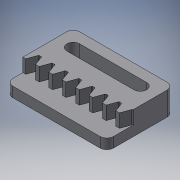
# Autodesk Inventor part: RackTest
Saved by Autodesk Inventor 2019 (Build 230136000, 136)
## iProperties
Created: 2019-07-15
Part Number: RackTest
Material: Generic
Document SubType Name: Modeling
Designer: aorfi
Density: 1 g/cm^3
Appearance: Default
Author: aorfi
Autodesk Inventor part; units mm, degrees
ref_plane "YZ Plane" through (0, 0, 0) normal (1, 0, 0) x (0, 1, 0)
ref_plane "XZ Plane" through (0, 0, 0) normal (0, 1, 0) x (-1, 0, 0)
ref_plane "XY Plane" through (0, 0, 0) normal (0, 0, 1) x (1, 0, 0)
sketch "Sketch1" plane through (0, 0, 0) normal (0, 1, 0) x (-1, 0, 0)
  line L0 (-15, 10) -> (15, 10)
  line L1 (15, 10) -> (15, -10)
  line L2 (15, -10) -> (-15, -10)
  line L3 (-15, -10) -> (-15, 10)
  line L4 (-15, 10) -> (15, -10) construction
  line L5 (15, 10) -> (-15, -10) construction
  circle A0 centre (10, -5) radius 1.8986
  circle A1 centre (-10, -5) radius 1.8986
  line L6 (10, -3.1013) -> (-10, -3.1013)
  line L7 (10, -6.8986) -> (-10, -6.8986)
  point P0 (0, 0)
  point P1 (0, 0)
  point P2 (10, 0)
  point P3 (0, 0)
  dimension "d0" = 30
  dimension "d1" = 20
  dimension "d8" = 5
  dimension "d61" = 3.7973
  dimension "d62" = 3.7973
  dimension "d63" = 5
  dimension "d64" = 5
  dimension "d67" = 5
  constraints: 16 end point, 4 midpoint, 4 point on circle, 3 tangent, 2 centre point, 2 horizontal, 2 horizontal alignment, 2 parallel, 1 perpendicular
  measures "d0" distance of L1.end L2.end
  measures "d1" distance of L0.end L1.end
  measures "d8" distance from line of L1 point (10, 0)
  measures "d61" diameter of A0
  measures "d62" diameter of A1
  measures "d63" distance from line of L2 A1.centre
  measures "d64" distance from line of A1.centre L3
  measures "d67" distance from line of L1 A0.centre
extrude "Extrusion1" add sketch "Sketch1" along normal mid plane 7
sketch "Sketch5" plane through (0, 3.5, 0) normal (0, -1, 0) x (1, 0, 0)
  arc A0 (10.771, 2.3227) -> (11.0102, 2.1552) centre (11.0102, 2.4098) ccw
  line L0 (11.0102, 2.1552) -> (11.5022, 2.1552)
  arc A1 (11.5022, 2.1552) -> (11.7414, 2.3227) centre (11.5022, 2.4098) ccw
  line L1 (11.7414, 2.3227) -> (12.7159, 5)
  line L2 (13.7863, 5) -> (12.7159, 5)
  line L3 (13.7863, 5) -> (14.7608, 2.3227)
  arc A2 (14.7608, 2.3227) -> (15, 2.1552) centre (15, 2.4098) ccw
  line L4 (11.5022, 2.4098) -> (15, 2.4098) construction
  line L5 (15, 10) -> (-15, 10) construction
  line L6 (15, -10) -> (15, 10) construction
  line L7 (10.771, 2.3227) -> (10.771, 10)
  line L8 (10.771, 10) -> (15, 10)
  line L9 (15, 10) -> (15, 2.1552)
  dimension "d49" = 0.2546
  dimension "d50" = 0.2546
  dimension "d51" = 0.4921
  dimension "d52" = 1.0704
  dimension "d53" = 2.8448
  dimension "d54" = 3.0194
  dimension "d55" = 0.2546
  dimension "d66" = 5
  constraints: 16 end point, 6 point on circle, 4 tangent, 3 centre point, 3 horizontal alignment, 2 collinear, 2 horizontal, 1 perpendicular, 1 point on line, 1 vertical
  measures "d49" radius of A0
  measures "d50" radius of A1
  measures "d51" distance of L0.start L0.end
  measures "d52" distance of L2.start L1.end
  measures "d53" distance between parallel lines of L2 L0
  measures "d54" distance of L3.end L1.start
  measures "d55" radius of A2
  measures "d66" distance between parallel lines of L8 L2
extrude "Extrusion4" cut sketch "Sketch5" along normal blind 3.5
pattern_linear "Rectangular Pattern1" count 10 spacing 3.99 along (-1, 0, 0) of "Extrusion4"
fillet "Fillet1" radius 2 4 edges at (-15, -1.75, 10) (15, -1.75, 10) (-15, 0, -10) (15, 0, -10)
equation "\"d62\" = d61"
equation "\"d67\" = d64"
equation "\"d55\" = d50"
body "Solid1"
